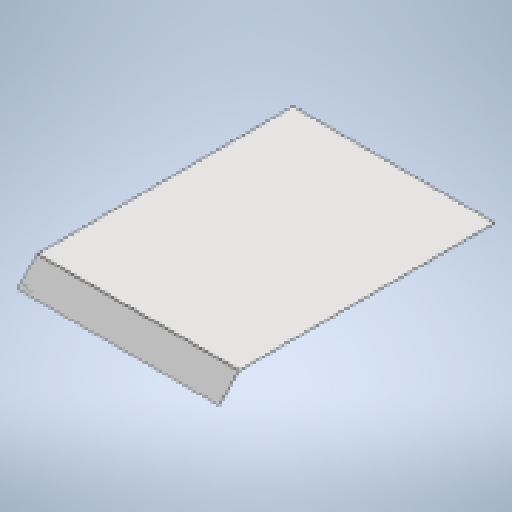
# Autodesk Inventor part: BSH 012 floor 2
Saved by Autodesk Inventor 2025 (Build 290162010, 162A)
## iProperties
Created: 2024-07-23
Part Number: BSH 012 floor 2
Material: 09g2s
Document SubType Name: Sheet Metal
Designer: admin
Mass: 81987.7 g
Surface Area: 69857.9 cm^2
Volume: 10444.3 cm^3
Density: 7.85 g/cm^3
Flat Pattern Width: 150 cm
Flat Pattern Length: 211.034 cm
Flat Pattern Area: 31655 cm^2
Sheet Metal Rule: AISI304 3mm Die 32
Sheet Metal Width: 1500,000 mm
Sheet Metal Length: 2110,336 mm
Sheet Metal Area: 3165504,449 mm^2
Appearance: Default
Author: admin
Autodesk Inventor part; units mm, degrees
ref_plane "YZ Plane" through (0, 0, 0) normal (1, 0, 0) x (0, 1, 0)
ref_plane "XZ Plane" through (0, 0, 0) normal (0, 1, 0) x (-1, 0, 0)
ref_plane "XY Plane" through (0, 0, 0) normal (0, 0, 1) x (1, 0, 0)
sketch "Sketch1" plane through (0, 0, 0) normal (0, 0, 1) x (1, 0, 0)
  line L0 (-750, -950) -> (750, -950)
  line L1 (750, -950) -> (750, 950)
  line L2 (750, 950) -> (-750, 950)
  line L3 (-750, 950) -> (-750, -950)
  line L4 (-750, -950) -> (750, 950) construction
  line L5 (750, -950) -> (-750, 950) construction
  point P0 (0, 0)
  dimension "d0" = 1500
  dimension "d1" = 1900
  measures "d0" distance of L2.end L1.end
  measures "d1" distance of L1.end L0.end
extrude "Plate1" add sketch "Sketch1" along normal blind 3
sketch "Sketch3" plane through (-750, -947.8787, 0.8787) normal (0, -0.7071068, 0.7071068) x (1, 0, 0)
  line L0 (1500, 0) -> (0, 0)
  line L1 (0, 0) -> (0, -212)
  line L2 (0, -212) -> (1500, -212)
  line L3 (1500, -212) -> (1500, 0)
  constraints: 6 end point, 1 horizontal, 1 perpendicular, 1 vertical
edge flange "Flange2" height 212 angle 45 thickness 3 bend radius 5 thickness toward (0, -0.7071068, 0.7071068) relief round relief width 3 relief depth 1.5 edges at (0, -950, 0) wall of the first edge with corners at (750, -947.8787, 0.8787) (-750, -947.8787, 0.8787) (-750, -1097.7853, -149.028) (750, -1097.7853, -149.028)
bend "Bend2"
corner "Corner2"
sketch "Sketch4" plane through (750, -1097.7853, -149.028) normal (0, 0.7071068, -0.7071068) x (-1, 0, 0)
  line L0 (1475, 36.661) -> (1475, 25) construction
  line L1 (1475, 25) -> (1275, 25) construction
  line L2 (1275, 25) -> (1275, 36.661) construction
  line L3 (1275, 36.661) -> (1475, 36.661) construction
  line L4 (0, 0) -> (1500, 0) projected
  line L5 (1500, 208.6863) -> (1500, 0) projected
  point P0 (750, 881.6301)
  point P1 (1475, 30.8305)
  dimension "d23" = 200
  dimension "d24" = 11.661
  dimension "d25" = 25
  dimension "d26" = 25
  constraints: 2 parallel, 1 midpoint, 2 other
  measures "d23" distance of L0.end L1.end
  measures "d24" distance between parallel lines of L1 L3
  measures "d25" distance between parallel lines of L4 L1
  measures "d26" distance from line of L5 point (1475, 30.83)
mark "Mark1"
equation "\"d2\" = Thickness"
equation "\"d13\" = BendReliefWidth"
equation "\"d14\" = BendReliefDepth"
equation "\"d15\" = MinimumRemnant"
equation "\"d16\" = TransitionRadius"
equation "\"d19\" = BendRadius"
equation "\"d20\" = CornerReliefSize"
equation "\"d21\" = GapSize"
equation "\"d22\" = JacobiRadiusSize"
equation "\"BendReliefWidth\" = Thickness"
equation "\"BendReliefDepth\" = 0.5 * Thickness"
equation "\"CornerReliefSize\" = 4 * Thickness"
equation "\"MinimumRemnant\" = 2 * Thickness"
equation "\"TransitionRadius\" = BendRadius"
equation "\"JacobiRadiusSize\" = BendRadius"
equation "\"GapSize\" = Thickness"
equation "\"Thickness\" = 3"
equation "\"BendRadius\" = 5"
body "Solid1"
